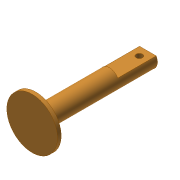
# Autodesk Inventor part: Front Axle
Saved by Autodesk Inventor 2016 (Build 200138000, 138)
## iProperties
Created: 2014-09-16
Part Number: Front Axle
Material: Generic
Document SubType Name: Modeling
Designer: loust
Density: 1 g/cm^3
Appearance: Default(2)
Author: loust
Autodesk Inventor part; units mm, degrees
ref_plane "YZ Plane" through (0, 0, 0) normal (1, 0, 0) x (0, 1, 0)
ref_plane "XZ Plane" through (0, 0, 0) normal (0, 1, 0) x (-1, 0, 0)
ref_plane "XY Plane" through (0, 0, 0) normal (0, 0, 1) x (1, 0, 0)
sketch "Sketch1" plane through (0, 0, 0) normal (0, 1, 0) x (-1, 0, 0)
  circle A0 centre (0, 0) radius 9.5
  dimension "d0" = 19
  constraints: 1 centre point, 1 coincident
  measures "d0" diameter of A0
extrude "Extrusion1" add sketch "Sketch1" along normal blind 1.4
sketch "Sketch2" plane through (0, 1.4, 0) normal (0, 1, 0) x (1, 0, 0)
  circle A0 centre (0, 0) radius 9.5 projected
  circle A1 centre (0, 0) radius 3.6
  dimension "d3" = 7.2
  constraints: 1 centre point, 1 coincident
  measures "d3" diameter of A1
extrude "Extrusion2" add sketch "Sketch2" along normal blind 42 contours A1
sketch "Sketch3" plane through (0, 43.4, 0) normal (0, 1, 0) x (1, 0, 0)
  circle A0 centre (0, 0) radius 3.6 projected
  line L0 (-3.1177, -1.8) -> (3.1177, -1.8)
  arc A1 (-3.1177, -1.8) -> (3.1177, -1.8) centre (0, 0) ccw
  dimension "d6" = 1.8
  constraints: 4 point on circle, 2 end point, 1 centre point, 1 coincident, 1 concentric, 1 horizontal
  measures "d6" distance from line of L0 A0.centre
extrude "Extrusion3" cut sketch "Sketch3" against normal blind 14.4 contours L0 A0 picked at (0.1393, -2.8389)
sketch "Sketch4" plane through (-3.1177, 43.4, 1.8) normal (0, 0, 1) x (1, 0, 0)
  line L0 (0, 0) -> (6.2354, 0) projected
  circle A0 centre (3.1177, -3.2) radius 1.2
  point P0 (3.1177, -43.4)
  dimension "d9" = 2.4
  dimension "d10" = 3.2
  constraints: 1 centre point
  measures "d9" diameter of A0
  measures "d10" distance from line of L0 A0.centre
extrude "Extrusion4" cut sketch "Sketch4" against normal through all
body "Solid1"
